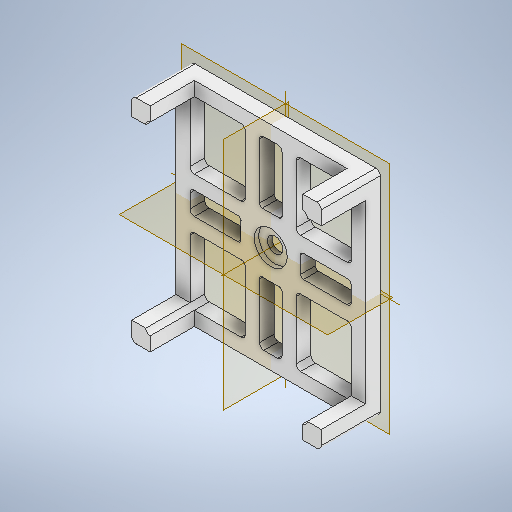
# Autodesk Inventor part: box-mount
Saved by Autodesk Inventor 2025.2 (Build 292293000, 293)
## iProperties
Created: 2025-04-08
Part Number: box-mount
Material: ABS Plastic
Document SubType Name: Modeling
Designer: yehorderehus
Density: 1.06 g/cm^3
Appearance: Smooth - White
Author: yehorderehus
Autodesk Inventor part; units mm, degrees
sketch "Sketch1" plane through (0, 0, 0) normal (0, 0, 1) x (1, 0, 0)
  line L0 (64.25, -72.25) -> (-64.25, -72.25)
  line L1 (-64.25, -72.25) -> (-64.25, 72.25)
  line L2 (-64.25, 72.25) -> (64.25, 72.25)
  line L3 (64.25, 72.25) -> (64.25, -72.25)
  circle A0 centre (0, 0) radius 5.2
  circle A1 centre (-59.5, -67.5) radius 1.25
  circle A2 centre (59.5, -67.5) radius 1.25
  circle A3 centre (59.5, 67.5) radius 1.25
  circle A4 centre (-59.5, 67.5) radius 1.25
  line L4 (-17.2, 72.25) -> (17.2, 72.25)
  line L5 (0, 101.15) -> (0, -101.15) projected
  line L6 (-54.75, 62.75) -> (-17.2, 62.75)
  line L7 (-17.2, 62.75) -> (-17.2, 17.2)
  line L8 (-17.2, 17.2) -> (-54.75, 17.2)
  line L9 (-54.75, 17.2) -> (-54.75, 62.75)
  line L10 (17.2, 17.2) -> (54.75, 17.2)
  line L11 (54.75, 17.2) -> (54.75, 62.75)
  line L12 (54.75, 62.75) -> (17.2, 62.75)
  line L13 (17.2, 62.75) -> (17.2, 17.2)
  line L14 (-17.2, -17.2) -> (-54.75, -17.2)
  line L15 (-54.75, -17.2) -> (-54.75, -62.75)
  line L16 (-54.75, -62.75) -> (-17.2, -62.75)
  line L17 (-17.2, -62.75) -> (-17.2, -17.2)
  line L18 (17.2, -17.2) -> (54.75, -17.2)
  line L19 (54.75, -17.2) -> (54.75, -62.75)
  line L20 (54.75, -62.75) -> (17.2, -62.75)
  line L21 (17.2, -62.75) -> (17.2, -17.2)
  line L22 (-89.95, 0) -> (89.95, 0) projected
  dimension "d0" = 10.4
  dimension "d12" = 119
  dimension "d14" = 135
  dimension "d44" = 3.5
  dimension "d45" = 3.5
  dimension "d46" = 3.5
  dimension "d47" = 3.5
  dimension "d48" = 3.5
  dimension "d49" = 3.5
  dimension "d50" = 12
  dimension "d51" = 12
  dimension "d52" = 3.5
  dimension "d53" = 67.5
  dimension "d54" = 2.5
  dimension "d55" = 59.5
  dimension "d56" = 12
  dimension "d57" = 3.5
  dimension "d58" = 12
  constraints: 42 end point, 10 equal length, 8 vertical alignment, 6 coincident, 6 horizontal, 5 centre point, 5 perpendicular, 4 horizontal alignment, 3 equal radius, 3 point on line
  measures "d0" diameter of A0
  measures "d12" distance of A1.centre A2.centre
  measures "d14" distance of A1.centre A4.centre
  measures "d44" distance edge to line of A1 L1
  measures "d45" distance edge to line of A1 L0
  measures "d46" distance edge to line of A4 L2
  measures "d47" distance edge to line of A2 L3
  measures "d48" distance edge to line of A1 L15
  measures "d49" distance edge to line of A2 L19
  measures "d50" distance edge to line of A0 L17
  measures "d51" distance edge to line of A0 L21
  measures "d52" distance edge to line of A1 L16
  measures "d53" distance from line of A1.centre L22
  measures "d54" diameter of A1
  measures "d55" distance from line of A1.centre L5
  measures "d56" distance edge to line of A0 L14
  measures "d57" distance edge to line of A4 L6
  measures "d58" distance edge to line of A0 L8
extrude "Extrusion1" add sketch "Sketch1" along normal blind 10 contours L0 L5 A0 L22 L3 | L0 L1 L22 A0 L5 | L22 A0 L5 L2 L3 | L5 L22 A0 | A0 L22 L5 | L22 L5 A0 | L1 L2 L5 A0 L22 | A0 L5 L22 | A1 | A2 | A3 | A4
fillet "Fillet1" radius 3 20 edges at (64.25, 72.25, 5) (-64.25, 72.25, 5) (64.25, -72.25, 5) (-64.25, -72.25, 5) (-54.75, 62.75, 5) (-17.2, 62.75, 5) (-17.2, 17.2, 5) (-54.75, 17.2, 5) (17.2, 62.75, 5) (54.75, 62.75, 5) (17.2, 17.2, 5) (54.75, 17.2, 5) (-17.2, -17.2, 5) (-54.75, -17.2, 5) (-17.2, -62.75, 5) (-54.75, -62.75, 5) (17.2, -62.75, 5) (17.2, -17.2, 5) (54.75, -17.2, 5) (54.75, -62.75, 5)
sketch "Sketch2" plane through (0, 0, 10) normal (0, 0, 1) x (1, 0, 0)
  line L0 (-89.95, 0) -> (89.95, 0) projected
  line L1 (0, 101.15) -> (0, -101.15) projected
  point P0 (0, 0)
  point P1 (0, 0)
  constraints: 1 coincident
hole "Hole2" at (0, 0, 10) direction (0, 0, -1) diameter 10.4 depth 10 counterbore diameter 22.4 counterbore depth 3
sketch "Sketch3" plane through (0, 0, 10) normal (0, 0, 1) x (1, 0, 0)
  arc A0 (-54.75, -59.75) -> (-51.75, -62.75) centre (-51.75, -59.75) ccw projected
  arc A1 (-51.75, 62.75) -> (-54.75, 59.75) centre (-51.75, 59.75) ccw projected
  arc A2 (54.75, 59.75) -> (51.75, 62.75) centre (51.75, 59.75) ccw projected
  arc A3 (64.25, 69.25) -> (61.25, 72.25) centre (61.25, 69.25) ccw projected
  arc A4 (-61.25, 72.25) -> (-64.25, 69.25) centre (-61.25, 69.25) ccw projected
  arc A5 (-64.25, -69.25) -> (-61.25, -72.25) centre (-61.25, -69.25) ccw projected
  arc A6 (61.25, -72.25) -> (64.25, -69.25) centre (61.25, -69.25) ccw projected
  arc A7 (51.75, -62.75) -> (54.75, -59.75) centre (51.75, -59.75) ccw projected
  line L0 (61.25, 72.25) -> (-61.25, 72.25) projected
  line L1 (-51.75, 72.25) -> (-51.75, 62.75)
  line L2 (-64.25, 69.25) -> (-64.25, -69.25) projected
  line L3 (-64.25, 59.75) -> (-54.75, 59.75)
  line L4 (-64.25, -59.75) -> (-54.75, -59.75)
  line L5 (-51.75, -72.25) -> (-51.75, -62.75)
  line L6 (-61.25, -72.25) -> (61.25, -72.25) projected
  line L7 (51.75, -72.25) -> (51.75, -62.75)
  line L8 (64.25, -59.75) -> (54.75, -59.75)
  line L9 (51.75, 72.25) -> (51.75, 62.75)
  line L10 (64.25, -69.25) -> (64.25, 69.25) projected
  line L11 (64.25, 59.75) -> (54.75, 59.75)
  line L12 (61.25, 72.25) -> (-61.25, 72.25) projected
  point P0 (0, 0)
  constraints: 16 end point, 8 point on line, 7 perpendicular, 1 horizontal
extrude "Extrusion2" add sketch "Sketch3" along normal blind 30 contours A0 L5 L6 A5 L2 L4 | L2 A4 L0 L1 A1 L3 | L7 A7 L8 L10 A6 L6 | L0 A3 L10 L11 A2 L9
sketch "Sketch4" plane through (0, 0, 0) normal (0, 0, -1) x (-1, 0, 0)
  line L0 (-15, 15) -> (15, 15)
  line L1 (15, 15) -> (15, -15)
  line L2 (15, -15) -> (-15, -15)
  line L3 (-15, -15) -> (-15, 15)
  line L4 (-19, 19) -> (19, 19) construction
  line L5 (19, 19) -> (19, -19) construction
  line L6 (19, -19) -> (-19, -19) construction
  line L7 (-19, -19) -> (-19, 19) construction
  line L8 (0, -101.15) -> (0, 101.15) projected
  line L9 (89.95, 0) -> (-89.95, 0) projected
  point P0 (0, 0)
  dimension "d92" = 30
  dimension "d93" = 30
  dimension "d94" = 4
  dimension "d95" = 4
  dimension "d96" = 4
  dimension "d97" = 4
  constraints: 16 end point, 4 parallel, 2 horizontal, 2 perpendicular, 2 other
  measures "d92" distance of L0.end L1.end
  measures "d93" distance of L0.start L0.end
  measures "d94" distance between parallel lines of L1 L5
  measures "d95" distance between parallel lines of L4 L0
  measures "d96" distance between parallel lines of L7 L3
  measures "d97" distance between parallel lines of L2 L6
extrude "Extrusion3" cut sketch "Sketch4" against normal blind 4
sketch "Sketch6" plane through (0, 0, 0) normal (0, 0, -1) x (-1, 0, 0)
  arc A0 (-54.75, 20.2) -> (-51.75, 17.2) centre (-51.75, 20.2) ccw projected
  line L0 (-51.75, 17.2) -> (-20.2, 17.2) projected
  line L1 (-54.75, 7.7) -> (-20.2, 7.7)
  line L2 (-20.2, 7.7) -> (-20.2, -7.7)
  line L3 (-20.2, -7.7) -> (-54.75, -7.7)
  line L4 (-54.75, -7.7) -> (-54.75, 7.7)
  line L5 (89.95, 0) -> (-89.95, 0) projected
  line L6 (20.2, 7.7) -> (54.75, 7.7)
  line L7 (54.75, 7.7) -> (54.75, -7.7)
  line L8 (54.75, -7.7) -> (20.2, -7.7)
  line L9 (20.2, -7.7) -> (20.2, 7.7)
  line L10 (20.2, 17.2) -> (51.75, 17.2) projected
  arc A1 (51.75, 17.2) -> (54.75, 20.2) centre (51.75, 20.2) ccw projected
  line L11 (-17.2, 20.2) -> (-17.2, 59.75) projected
  arc A2 (-17.2, 59.75) -> (-20.2, 62.75) centre (-20.2, 59.75) ccw projected
  line L12 (-17.2, -59.75) -> (-17.2, -20.2) projected
  arc A3 (-20.2, -62.75) -> (-17.2, -59.75) centre (-20.2, -59.75) ccw projected
  line L13 (-7.7, -20.2) -> (7.7, -20.2)
  line L14 (7.7, -20.2) -> (7.7, -62.75)
  line L15 (7.7, -62.75) -> (-7.7, -62.75)
  line L16 (-7.7, -62.75) -> (-7.7, -20.2)
  line L17 (0, -101.15) -> (0, 101.15) projected
  line L18 (-7.7, 20.2) -> (7.7, 20.2)
  line L19 (7.7, 20.2) -> (7.7, 62.75)
  line L20 (7.7, 62.75) -> (-7.7, 62.75)
  line L21 (-7.7, 62.75) -> (-7.7, 20.2)
  point P0 (0, 0)
  dimension "d102" = 9.5
  dimension "d103" = 9.5
  constraints: 32 end point, 8 parallel, 6 horizontal alignment, 6 vertical alignment, 4 horizontal, 4 perpendicular, 2 other
  measures "d102" distance between parallel lines of L0 L1
  measures "d103" distance between parallel lines of L12 L16
extrude "Extrusion4" cut sketch "Sketch6" against normal through all
fillet "Fillet3" radius 2 8 edges at (20.2, -7.7, 5) (20.2, 7.7, 5) (7.7, -20.2, 5) (-7.7, -20.2, 5) (-20.2, -7.7, 5) (-20.2, 7.7, 5) (-7.7, 20.2, 5) (7.7, 20.2, 5)
fillet "Fillet4" radius 3 8 edges at (-7.7, 62.75, 5) (7.7, 62.75, 5) (-54.75, 7.7, 5) (-54.75, -7.7, 5) (-7.7, -62.75, 5) (7.7, -62.75, 5) (54.75, -7.7, 5) (54.75, 7.7, 5)
equation "\"d46\" = d45"
equation "\"d47\" = d44"
equation "\"d48\" = d44"
equation "\"d49\" = d44"
equation "\"d52\" = d45"
equation "\"d53\" = 0.5 * d14"
equation "\"d55\" = 0.5 * d12"
body "Solid1"
